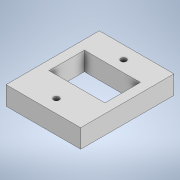
# Autodesk Inventor part: AdaptadorSensorInductivoV3
Saved by Autodesk Inventor 2020.3 (Build 243373000, 373)
## iProperties
Created: 2020-09-23
Part Number: AdaptadorSensorInductivoV3
Material: Generic
Document SubType Name: Modeling
Designer: mifer
Density: 1 g/cm^3
Appearance: Default
Author: mifer
## iProperties of the stored document _3DPrint.ipt
Created: 2020-09-23
Part Number: _3DPrint
Material: Generic
Document SubType Name: Modeling
Designer: mifer
Density: 1 g/cm^3
Appearance: Default
Author: mifer
Autodesk Inventor part; units mm, degrees
ref_plane "YZ Plane" through (0, 0, 0) normal (1, 0, 0) x (0, 1, 0)
ref_plane "XZ Plane" through (0, 0, 0) normal (0, 1, 0) x (-1, 0, 0)
ref_plane "XY Plane" through (0, 0, 0) normal (0, 0, 1) x (1, 0, 0)
sketch "Sketch1" plane through (0, 0, 0) normal (0, 1, 0) x (-1, 0, 0)
  line L0 (0, 0) -> (40, 0)
  line L1 (40, 0) -> (40, -50)
  line L2 (40, -50) -> (0, -50)
  line L3 (0, -50) -> (0, 0)
  line L4 (40, 0) -> (0, 0)
  line L5 (0, 0) -> (0, -18)
  line L6 (5, -18) -> (35, -18)
  line L7 (40, -18) -> (40, 0)
  line L8 (35, -18) -> (5, -18)
  line L9 (0, -18) -> (0, -37)
  line L10 (5, -37) -> (35, -37)
  line L11 (40, -37) -> (40, -18)
  circle A0 centre (20, -7) radius 1.5
  circle A1 centre (20, -43) radius 1.5
  line L12 (20, -18) -> (35, -18)
  line L13 (35, -18) -> (35, -37)
  line L14 (35, -37) -> (20, -37)
  line L15 (20, -37) -> (5, -37)
  line L16 (5, -37) -> (5, -18)
  line L17 (5, -18) -> (20, -18)
  dimension "d0" = 40
  dimension "d1" = 50
  dimension "d2" = 3
  dimension "d3" = 3
  constraints: 36 end point, 8 parallel, 5 horizontal, 5 perpendicular, 2 centre point, 2 point on line, 1 midpoint
  measures "d0" distance of L1.end L2.end
  measures "d1" distance of L0.end L1.end
  measures "d2" diameter of A0
  measures "d3" diameter of A1
extrude "Extrusion1" add sketch "Sketch1" along normal blind 10
body "Solid1"
